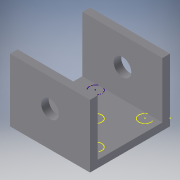
# Autodesk Inventor part: channel1 of lift pivot
Saved by Autodesk Inventor 2016 (Build 200138000, 138)
## iProperties
Created: 2015-11-14
Part Number: channel1 of lift pivot
Material: Generic
Document SubType Name: Modeling
Designer: jesse
Density: 1 g/cm^3
Appearance: Default
Author: jesse
Autodesk Inventor part; units mm, degrees
ref_plane "YZ Plane" through (0, 0, 0) normal (1, 0, 0) x (0, 1, 0)
ref_plane "XZ Plane" through (0, 0, 0) normal (0, 1, 0) x (-1, 0, 0)
ref_plane "XY Plane" through (0, 0, 0) normal (0, 0, 1) x (1, 0, 0)
sketch "Sketch1" plane through (0, 0, 0) normal (0, 1, 0) x (-1, 0, 0)
  line L0 (16.1798, 16.1798) -> (0, 16.1798)
  line L1 (0, 16.1798) -> (0, 0)
  line L2 (0, 0) -> (16.1798, 0)
  line L3 (16.1798, 0) -> (16.1798, 16.1798)
  dimension "d0" = 16.1798
  dimension "d1" = 16.1798
  constraints: 8 end point, 2 parallel, 1 horizontal, 1 perpendicular
  measures "d0" distance of L2.end L0.start
  measures "d1" distance of L0.start L0.end
extrude "Extrusion1" add sketch "Sketch1" along normal blind 1.4478
sketch "Sketch2" plane through (0, 1.4478, 0) normal (0, 1, 0) x (1, 0, 0)
  line L0 (0, -16.1798) -> (0, 0) projected
  line L1 (-16.1798, 0) -> (-16.1798, -16.1798) projected
  line L2 (0, 0) -> (-16.1798, 0)
  line L3 (-16.1798, 0) -> (-16.1798, -1.524)
  line L4 (-16.1798, -1.524) -> (0, -1.524)
  line L5 (0, -1.524) -> (0, 0)
  line L6 (-16.1798, -16.1798) -> (0, -16.1798)
  line L7 (0, -16.1798) -> (0, -14.6558)
  line L8 (0, -14.6558) -> (-16.1798, -14.6558)
  line L9 (-16.1798, -14.6558) -> (-16.1798, -16.1798)
  dimension "d4" = 1.524
  dimension "d5" = 1.524
  constraints: 16 end point, 4 parallel, 2 horizontal, 2 perpendicular, 2 point on line
  measures "d4" distance between parallel lines of L2 L4
  measures "d5" distance between parallel lines of L6 L8
extrude "Extrusion2" add sketch "Sketch2" along normal blind 11.2776 contours L6 L1 L8 L0 | L4 L1 L2 L0
sketch "Sketch3" plane through (-16.1798, 0, 16.1798) normal (0, 0, 1) x (1, 0, 0)
  circle A0 centre (8.0899, 7.0866) radius 1.7859
  line L0 (0, 1.4478) -> (0, 12.7254) construction
  line L1 (0, 7.0866) -> (16.1798, 7.0866) construction
  line L2 (16.1798, 1.4478) -> (16.1798, 12.7254) construction
  line L3 (16.1798, 12.7254) -> (0, 12.7254) construction
  line L4 (8.0899, 12.7254) -> (8.0899, 0) construction
  line L5 (0, 0) -> (16.1798, 0) construction
  dimension "d8" = 3.5719
  constraints: 5 midpoint, 4 end point, 1 centre point, 1 point on line
  measures "d8" diameter of A0
extrude "Extrusion3" cut sketch "Sketch3" against normal through all
sketch "Sketch4" plane through (0, 1.4478, 0) normal (0, 1, 0) x (1, 0, 0)
  circle A0 centre (-7.7025, -8.3571) radius 1.25 projected
  arc A1 (-13.8611, -2.8949) -> (-13.1534, -2.1884) centre (-12.6979, -3.3525) ccw projected
  arc A2 (-2.2403, -2.1985) -> (-1.5338, -2.9063) centre (-2.6979, -3.3617) ccw projected
  arc A3 (-1.5439, -13.8193) -> (-2.2517, -14.5258) centre (-2.7072, -13.3617) ccw projected
  arc A4 (-13.1648, -14.5157) -> (-13.8712, -13.8079) centre (-12.7072, -13.3525) ccw projected
  circle A5 centre (-12.7072, -13.3525) radius 1.25
  circle A6 centre (-12.6979, -3.3525) radius 1.25
  circle A7 centre (-12.6979, -3.3525) radius 1.25
  circle A8 centre (-2.7072, -13.3617) radius 1.25
  circle A9 centre (-2.6979, -3.3617) radius 1.25
  point P0 (0, 0)
  constraints: 5 centre point, 5 coincident, 3 concentric
extrude "Extrusion4" cut sketch "Sketch4" against normal through all
body "Solid1"
